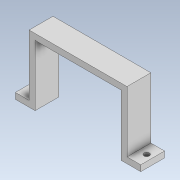
# Autodesk Inventor part: battery_fix
Saved by Autodesk Inventor 2020 (Build 240168000, 168)
## iProperties
Created: 2021-02-09
Part Number: battery_fix
Material: Generic
Document SubType Name: Modeling
Designer: DELL
Density: 1 g/cm^3
Appearance: Default
Author: DELL
Autodesk Inventor part; units mm, degrees
ref_plane "YZ Plane" through (0, 0, 0) normal (1, 0, 0) x (0, 1, 0)
ref_plane "XZ Plane" through (0, 0, 0) normal (0, 1, 0) x (-1, 0, 0)
ref_plane "XY Plane" through (0, 0, 0) normal (0, 0, 1) x (1, 0, 0)
sketch "Sketch1" plane through (0, 0, 0) normal (0, 0, 1) x (1, 0, 0)
  line L0 (-52.5, 5) -> (-41, 5)
  line L1 (-41, 5) -> (-41, 56)
  line L2 (-41, 56) -> (41, 56)
  line L3 (41, 56) -> (41, 5)
  line L4 (41, 5) -> (52.5, 5)
  line L5 (-36, 0) -> (-36, 51)
  line L6 (-36, 51) -> (36, 51)
  line L7 (36, 51) -> (36, 0)
  line L8 (0, 0) -> (0, -25.7238) construction
  line L9 (52.5, 0) -> (52.5, 5)
  line L10 (-52.5, 0) -> (-52.5, 5)
  line L11 (-52.5, 0) -> (-36, 0)
  line L12 (36, 0) -> (52.5, 0)
  dimension "d1" = 5
  dimension "d2" = 5
  dimension "d3" = 5
  dimension "d5" = 72
  dimension "d6" = 51
  dimension "d7" = 16.5
  dimension "d8" = 5
  constraints: 26 end point, 4 perpendicular, 3 horizontal, 3 point on line, 2 equal length, 1 collinear, 1 vertical, 2 other
  measures "d1" distance between parallel lines of L1 L5
  measures "d2" distance between parallel lines of L2 L6
  measures "d3" distance between parallel lines of L3 L7
  measures "d5" distance between parallel lines of L7 L5
  measures "d6" distance between parallel lines of L6 L11
  measures "d7" distance between parallel lines of L10 L5
  measures "d8" distance between parallel lines of L11 L0
extrude "Extrusion1" add sketch "Sketch1" along normal mid plane 20
sketch "Sketch2" plane through (-52.5, 0, 10) normal (0, -1, 0) x (1, 0, 0)
  circle A0 centre (5, -10) radius 1.25
  circle A1 centre (100, -10) radius 1.25
  line L0 (52.5, -10) -> (52.5, 0) construction
  line L1 (16.5, 0) -> (88.5, 0) construction
  circle A2 centre (5, -10) radius 2.25
  circle A3 centre (100, -10) radius 2.25
  dimension "d11" = 2.5
  dimension "d12" = 95
  dimension "d15" = 4.5
  constraints: 4 centre point, 2 coincident, 2 end point, 2 equal radius, 2 horizontal alignment, 1 midpoint, 1 symmetric about line
  measures "d11" diameter of A0
  measures "d12" distance of A1.centre A0.centre
  measures "d15" diameter of A3
extrude "Extrusion2" cut sketch "Sketch2" against normal through all contours A0 | A1
extrude "Extrusion3" cut sketch "Sketch2" along normal blind 3 from surface at -5
equation "\"d1\" = d8"
equation "\"d2\" = d8"
equation "\"d3\" = d8"
body "Solid1"
